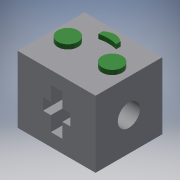
# Autodesk Inventor part: head
Saved by Autodesk Inventor 2019 (Build 230136000, 136)
## iProperties
Created: 2018-05-20
Part Number: head
Material: 一般
Document SubType Name: Modeling
Designer: uctom
Density: 1 g/cm^3
Appearance: 既定
Author: uctom
Autodesk Inventor part; units mm, degrees
ref_plane "YZ Plane" through (0, 0, 0) normal (1, 0, 0) x (0, 1, 0)
ref_plane "XZ Plane" through (0, 0, 0) normal (0, 1, 0) x (-1, 0, 0)
ref_plane "XY Plane" through (0, 0, 0) normal (0, 0, 1) x (1, 0, 0)
sketch "スケッチ1" plane through (0, 0, 0) normal (0, 0, 1) x (1, 0, 0)
  line L0 (40.6372, 0) -> (-44.8968, 0)
  line L1 (0, -28.7297) -> (0, 26.7749)
  line L2 (17.5, -15) -> (-17.5, -15)
  line L3 (-17.5, -15) -> (-17.5, 15)
  line L4 (-17.5, 15) -> (17.5, 15)
  line L5 (17.5, 15) -> (17.5, -15)
  point P0 (0, 0)
  dimension "d0" = 35
  dimension "d1" = 30
  constraints: 12 end point, 2 horizontal, 2 parallel, 2 point on line, 1 perpendicular, 1 vertical, 2 other
  measures "d0" distance of L3.end L4.end
  measures "d1" distance of L2.end L3.end
extrude "押し出し1" add sketch "スケッチ1" along normal blind 30
sketch "スケッチ4" plane through (17.5, -15, 0) normal (1, 0, 0) x (0, 0, -1)
  line L0 (0, 30) -> (0, 0) projected
  line L1 (0, 30) -> (-30, 30) projected
  line L2 (-30, 0) -> (-30, 30) projected
  line L3 (0, 0) -> (-30, 0) projected
  line L4 (-30, 15) -> (0, 15)
  line L5 (0, 30) -> (-30, 30) projected
  line L6 (-15, 30) -> (-15, 0)
  circle A0 centre (-15, 15) radius 5
  dimension "d4" = 10
  constraints: 4 end point, 4 midpoint, 1 centre point, 1 horizontal
  measures "d4" diameter of A0
extrude "押し出し2" cut sketch "スケッチ4" against normal through all contours A0 L6 L4 | L4 L6 A0 | L6 L4 A0 | L6 A0 L4
sketch "スケッチ5" plane through (0, 0, 30) normal (0, 0, 1) x (1, 0, 0)
  line L0 (-5.9, -2.4) -> (-5.9, 2.4) projected
  line L1 (-2.4, -2.4) -> (-5.9, -2.4) projected
  line L2 (-2.4, -9) -> (-2.4, -2.4) projected
  line L3 (2.4, -9) -> (-2.4, -9) projected
  line L4 (2.4, -2.4) -> (2.4, -9) projected
  line L5 (5.9, -2.4) -> (2.4, -2.4) projected
  line L6 (5.9, 2.4) -> (5.9, -2.4) projected
  line L7 (2.4, 2.4) -> (5.9, 2.4) projected
  line L8 (2.4, 9) -> (2.4, 2.4) projected
  line L9 (-2.4, 9) -> (2.4, 9) projected
  line L10 (-2.4, 2.4) -> (-2.4, 9) projected
  line L11 (-5.9, 2.4) -> (-2.4, 2.4) projected
  ellipse E0 centre (0.5, 0) end of major axis (4.0355, 0) minor radius 2.5 (0, -2.4749) -> (0, 2.4749) ccw projected
  ellipse E1 centre (-0.5, 0) end of major axis (-4.0355, 0) minor radius 2.5 (0, 2.4749) -> (0, -2.4749) ccw projected
  line L12 (-2.6, 9.2) -> (2.6, 9.2)
  line L13 (2.6, 9.2) -> (2.6, 2.6)
  line L14 (2.6, 2.6) -> (6.1, 2.6)
  line L15 (6.1, 2.6) -> (6.1, -2.6)
  line L16 (6.1, -2.6) -> (2.6, -2.6)
  line L17 (2.6, -2.6) -> (2.6, -9.2)
  line L18 (2.6, -9.2) -> (-2.6, -9.2)
  line L19 (-2.6, -9.2) -> (-2.6, -2.6)
  line L20 (-2.6, -2.6) -> (-6.1, -2.6)
  line L21 (-6.1, -2.6) -> (-6.1, 2.6)
  line L22 (-6.1, 2.6) -> (-2.6, 2.6)
  line L23 (-2.6, 2.6) -> (-2.6, 9.2)
  point P0 (0, 0)
  dimension "d9" = 0.2
  constraints: 24 end point, 13 other
  measures "d9" distance between parallel lines of L10 L23
extrude "押し出し3" cut sketch "スケッチ5" against normal up to surface (30 mm away) contours L0 L11 L10 L9 L8 L7 L6 L5 L4 L3 L2 L1 | E1 E0 | L12 L13 L14 L15 L16 L17 L18 L19 L20 L21 L22 L23
sketch "スケッチ6" plane through (-17.5, 15, 0) normal (0, 1, 0) x (1, 0, 0)
  line L0 (0, 0) -> (35, 0) projected
  line L1 (0, 0) -> (0, -30) projected
  line L2 (35, -30) -> (0, -30) projected
  line L3 (35, 0) -> (35, -30) projected
  line L4 (35, -10) -> (35, -20) projected
  line L5 (35, -15) -> (0, -15)
  line L6 (0, -30) -> (35, -30) projected
  line L7 (17.5, -30) -> (17.5, 0)
  circle A0 centre (7.5246, -15) radius 4.5427
  line L8 (21.5, -7.2467) -> (17.5, -6.2467) construction
  line L9 (17.5, -6.2467) -> (13.5, -7.2467) construction
  spline S0 degree 2 poles (21.5, -7.2467) (17.5, -6.2467) (13.5, -7.2467) knots 1 1 1 2 2 2
  line L10 (21.5, -7.2467) -> (21.5, -5.2467)
  line L11 (21.5, -5.2467) -> (17.5, -2.1432) construction
  line L12 (17.5, -2.1432) -> (13.5, -5.2467) construction
  spline S1 degree 2 poles (21.5, -5.2467) (17.5, -2.1432) (13.5, -5.2467) knots 1 1 1 2 2 2
  line L13 (13.5, -5.2467) -> (13.5, -7.2467)
  circle A1 centre (27.4754, -15) radius 4.5427
  line L14 (13.5, -7.2467) -> (29.7216, -7.2467)
  line L15 (13.5, -5.2467) -> (30.3964, -5.2467)
  dimension "d12" = 2
  dimension "d13" = 4
  dimension "d14" = 4
  constraints: 12 end point, 5 point on line, 3 midpoint, 3 vertical, 2 centre point, 2 horizontal, 1 symmetric about line, 7 other
  measures "d12" distance of L12.end L9.end
  measures "d13" distance between parallel lines of L13 L7
  measures "d14" distance between parallel lines of L10 L7
extrude "顔" add sketch "スケッチ6" along normal blind 2 contours S1 L15 L7 | L7 L15 S1 | A0 L5 | L5 A0 | L15 L10 S0 L7 | L7 S0 L13 L15 | A1 L5 | L5 A1
equation "\"d14\" = d13"
